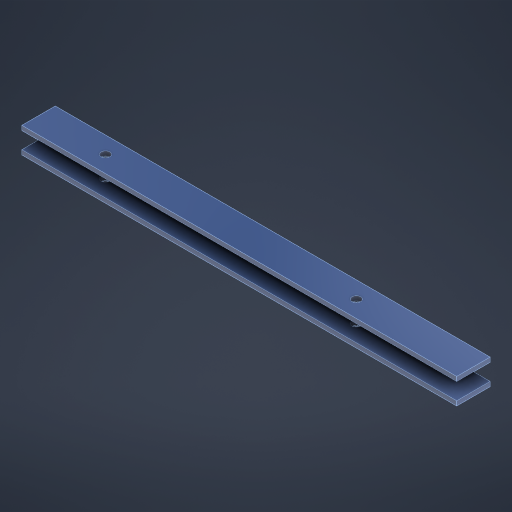
# Autodesk Inventor part: ArmPart2Mini
Saved by Autodesk Inventor 2024.2 (Build 282272000, 272)
## iProperties
Created: 2024-01-04
Part Number: ArmPart2Mini
Material: Generic
Document SubType Name: Modeling
Designer: student
Density: 1 g/cm^3
Appearance: Flaked Satin - Blue
Author: student
Autodesk Inventor part; units mm, degrees
ref_plane "YZ Plane" through (0, 0, 0) normal (1, 0, 0) x (0, 1, 0)
ref_plane "XZ Plane" through (0, 0, 0) normal (0, 1, 0) x (-1, 0, 0)
ref_plane "XY Plane" through (0, 0, 0) normal (0, 0, 1) x (1, 0, 0)
sketch "Sketch1" plane through (0, 0, 0) normal (0, 1, 0) x (-1, 0, 0)
  line L0 (0, 0) -> (431.8, 0)
  line L1 (431.8, 0) -> (431.8, -25.4)
  line L2 (431.8, -25.4) -> (0, -25.4)
  line L3 (0, -25.4) -> (0, 0)
  dimension "d0" = 431.8
  dimension "d1" = 25.4
  constraints: 8 end point, 2 parallel, 1 horizontal, 1 perpendicular
  measures "d0" distance of L1.end L2.end
  measures "d1" distance of L0.end L1.end
extrude "Extrusion1" add sketch "Sketch1" along normal blind 3.429
sketch "Sketch2" plane through (0, 3.429, 0) normal (0, 1, 0) x (1, 0, 0)
  line L0 (0, 25.4) -> (-431.8, 25.4) projected
  line L1 (-44.45, 25.4) -> (-171.0436, 25.4)
  line L2 (-171.0436, 25.4) -> (-171.0436, 21.7932)
  line L3 (-171.0436, 21.7932) -> (-44.45, 21.7932)
  line L4 (-44.45, 21.7932) -> (-44.45, 25.4)
  line L5 (0, 0) -> (0, 25.4) projected
  point P0 (-44.45, 23.5966)
  dimension "d4" = 126.5936
  dimension "d5" = 3.6068
  dimension "d6" = 44.45
  constraints: 8 end point, 2 parallel, 1 horizontal, 1 midpoint, 1 perpendicular, 1 point on line
  measures "d4" distance of L3.end L2.end
  measures "d5" distance of L2.end L1.end
  measures "d6" distance from line of L5 point (-44.45, 23.597)
extrude "Extrusion2" add sketch "Sketch2" along normal blind 12.5984
sketch "Sketch3" plane through (0, 16.0274, 0) normal (0, 1, 0) x (1, 0, 0)
  line L0 (-431.8, 0) -> (0, 0)
  line L1 (0, 0) -> (0, 25.4)
  line L2 (0, 25.4) -> (-431.8, 25.4)
  line L3 (-431.8, 25.4) -> (-431.8, 0)
  constraints: 8 end point, 2 parallel, 1 horizontal, 1 perpendicular
extrude "Extrusion3" add sketch "Sketch3" along normal blind 3.429
sketch "Sketch4" plane through (0, 19.4564, 0) normal (0, 1, 0) x (1, 0, 0)
  line L0 (0, 25.4) -> (-431.8, 25.4) projected
  line L1 (0, 0) -> (0, 25.4) projected
  line L2 (-431.8, 25.4) -> (-431.8, 0) projected
  point P0 (-12.7, 12.7)
  point P1 (-419.1, 12.7)
  point P2 (-203.2, 12.7)
  dimension "d11" = 12.7
  dimension "d12" = 12.7
  dimension "d13" = 12.7
  dimension "d14" = 12.7
  dimension "d15" = 12.7
  dimension "d16" = 203.2
  measures "d11" distance from line of L0 point (-12.7, 12.7)
  measures "d12" distance from line of L1 point (-12.7, 12.7)
  measures "d13" distance from line of L2 point (-419.1, 12.7)
  measures "d14" distance from line of L0 point (-419.1, 12.7)
  measures "d15" distance from line of L0 point (-203.2, 12.7)
  measures "d16" distance from line of L1 point (-203.2, 12.7)
hole "Hole1" at (-12.7, 19.4564, -12.7) at (-203.2, 19.4564, -12.7) direction (0, -1, 0) diameter 6.5024 end through all
sketch "Sketch6" plane through (0, 0, 0) normal (0, -1, 0) x (1, 0, 0)
  circle A0 centre (-203.2, -12.7) radius 3.2512 projected
  circle A1 centre (-12.7, -12.7) radius 3.2512 projected
  line L0 (0, -25.4) -> (-431.8, -25.4) projected
  line L1 (0, 0) -> (0, -25.4) projected
  line L2 (-431.8, 0) -> (0, 0) projected
  line L3 (-431.8, -25.4) -> (-431.8, 0) projected
  line L4 (-431.8, -25.4) -> (-254, -25.4)
  line L5 (-254, -25.4) -> (-254, 0)
  line L6 (-254, 0) -> (-431.8, 0)
  line L7 (-431.8, 0) -> (-431.8, -25.4)
  dimension "d26" = 177.8
  constraints: 8 end point, 2 parallel, 1 horizontal, 1 perpendicular, 1 point on line
  measures "d26" distance of L6.end L5.end
extrude "Extrusion5" cut sketch "Sketch6" against normal blind 76.2 contours L0 L3 L2 L5
sketch "Sketch7" plane through (0, 0, 0) normal (1, 0, 0) x (0, 0, -1)
  line L0 (0, 0) -> (25.4, 0) projected
  line L1 (25.4, 0) -> (25.4, 3.429) projected
  line L2 (0, 3.429) -> (25.4, 3.429) projected
  line L3 (0, 0) -> (0, 3.429) projected
  line L4 (0, 16.0274) -> (25.4, 16.0274) projected
  line L5 (25.4, 16.0274) -> (25.4, 19.4564) projected
  line L6 (0, 19.4564) -> (25.4, 19.4564) projected
  line L7 (0, 16.0274) -> (0, 19.4564) projected
extrude "Extrusion6" add sketch "Sketch7" along normal blind 76.2
body "Solid1"
